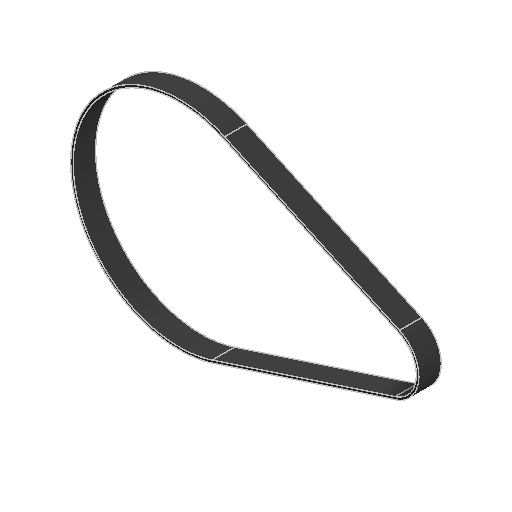
# Autodesk Inventor part: Diff Motor Belts
Saved by Autodesk Inventor 2025.2 (Build 292293000, 293)
## iProperties
Created: 2025-02-20
Part Number: Diff Motor Belts
Material: Generic
Document SubType Name: Modeling
Designer: Jakeg
Density: 1 g/cm^3
Appearance: Default
Author: Jakeg
Autodesk Inventor part; units mm, degrees
ref_plane "YZ Plane" through (0, 0, 0) normal (1, 0, 0) x (0, 1, 0)
ref_plane "XZ Plane" through (0, 0, 0) normal (0, 1, 0) x (-1, 0, 0)
ref_plane "XY Plane" through (0, 0, 0) normal (0, 0, 1) x (1, 0, 0)
sketch "Sketch1" plane through (0, 0, 0) normal (0, 0, 1) x (1, 0, 0)
  circle A0 centre (0, 0) radius 43.0276
  circle A1 centre (83.6836, -4.7804) radius 12.4968
  circle A2 centre (0, 0) radius 44.0436
  circle A3 centre (83.6836, -4.7804) radius 13.5128
  line L0 (13.6771, -41.8662) -> (87.8798, -17.6251)
  line L1 (13.3616, -40.9004) -> (87.5643, -16.6593)
  line L2 (88.8918, 6.5794) -> (17.9323, 39.1127)
  line L3 (89.3152, 7.503) -> (18.3557, 40.0363)
  point P0 (17.6469, -33.9959)
  point P1 (17.4567, 34.094)
  dimension "d0" = 86.0552
  dimension "d1" = 24.9936
  dimension "d2" = 83.82
  dimension "d3" = 88.0872
  dimension "d4" = 27.0256
  dimension "d5" = 1.016
  dimension "d6" = 1.016
  constraints: 8 end point, 8 point on circle, 4 centre point, 4 tangent, 3 coincident, 2 parallel
  measures "d0" diameter of A0
  measures "d1" diameter of A1
  measures "d2" distance of A1.centre point (0, 0)
  measures "d3" diameter of A2
  measures "d4" diameter of A3
  measures "d5" distance between parallel lines of L3 L2
  measures "d6" distance between parallel lines of L1 L0
extrude "Extrusion1" add sketch "Sketch1" along normal blind 9.0932 contours A0 L1 A2 L2 | A2 L3 A3 L2 | L1 A3 L0 A2 | A3 L1 A1 L2 picked at (-23.5196, -36.5948) picked at (90.0516, 6.6643)
body "Solid1"
